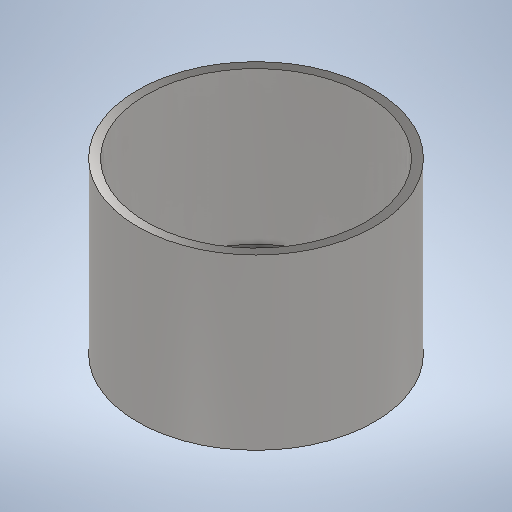
# Autodesk Inventor part: Gelenk 2
Saved by Autodesk Inventor 2025.2 (Build 292293000, 293)
## iProperties
Created: 2025-05-16
Part Number: Gelenk 2
Material: Steel, Alloy
Document SubType Name: Modeling
Designer: MSIGAMING
Mass: 6435.4 g
Surface Area: 1030.44 cm^2
Volume: 832.522 cm^3
Density: 7.73 g/cm^3
Appearance: Semi-Polished
Author: MSIGAMING
Autodesk Inventor part; units mm, degrees
ref_plane "YZ Plane" through (0, 0, 0) normal (1, 0, 0) x (0, 1, 0)
ref_plane "XZ Plane" through (0, 0, 0) normal (0, 1, 0) x (-1, 0, 0)
ref_plane "XY Plane" through (0, 0, 0) normal (0, 0, 1) x (1, 0, 0)
sketch "Sketch1" plane through (0, 0, 0) normal (0, 1, 0) x (-1, 0, 0)
  circle A0 centre (0, 0) radius 70
  circle A1 centre (0, 0) radius 65
  dimension "d0" = 140
  dimension "d1" = 130
  constraints: 2 centre point, 2 coincident
  measures "d0" diameter of A0
  measures "d1" diameter of A1
extrude "Extrusion1" add sketch "Sketch1" along normal mid plane 100
sketch "Sketch6" plane through (0, -50, 0) normal (0, -1, 0) x (1, 0, 0)
  circle A0 centre (0, 0) radius 70 projected
extrude "Extrusion5" add sketch "Sketch6" against normal blind 10
body "Solid1"
